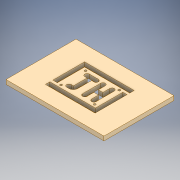
# Autodesk Inventor part: JH
Saved by Autodesk Inventor 2017 (Build 210142000, 142)
## iProperties
Created: 2016-09-28
Part Number: JH
Material: Polyethylene, High Density
Document SubType Name: Modeling
Designer: jhaun
Density: 0.952 g/cm^3
Appearance: Smooth - Off-White
Author: jhaun
Autodesk Inventor part; units mm, degrees
ref_plane "YZ Plane" through (0, 0, 0) normal (1, 0, 0) x (0, 1, 0)
ref_plane "XZ Plane" through (0, 0, 0) normal (0, 1, 0) x (-1, 0, 0)
ref_plane "XY Plane" through (0, 0, 0) normal (0, 0, 1) x (1, 0, 0)
sketch "Sketch1" plane through (0, 0, 0) normal (0, 0, 1) x (1, 0, 0)
  arc A0 (0, 6.5) -> (0, -6.5) centre (0, 0) ccw
  line L0 (0, 6.5) -> (26, 6.5)
  line L1 (0, -6.5) -> (6.5, -6.5)
  arc A1 (26, -6.5) -> (26, 6.5) centre (26, 0) ccw
  line L2 (26, -6.5) -> (19.5, -6.5)
  line L3 (6.5, -6.5) -> (6.5, -45.5)
  line L4 (19.5, -6.5) -> (19.5, -45.5)
  line L5 (6.5, -45.5) -> (0, -45.5)
  arc A2 (0, -45.5) -> (0, -58.5) centre (0, -52) ccw
  line L6 (0, -58.5) -> (6.5, -58.5)
  arc A3 (6.5, -58.5) -> (19.5, -45.5) centre (6.5, -45.5) ccw
  line L7 (39, 0) -> (39, -52)
  arc A4 (39, -52) -> (52, -52) centre (45.5, -52) ccw
  line L8 (52, -52) -> (52, -32.5)
  line L9 (52, -32.5) -> (65, -32.5)
  line L10 (65, 0) -> (65, -19.5)
  line L11 (65, -19.5) -> (52, -19.5)
  line L12 (52, -19.5) -> (52, 0)
  line L13 (78, 0) -> (78, -52)
  line L14 (65, -32.5) -> (65, -52)
  arc A5 (65, -52) -> (78, -52) centre (71.5, -52) ccw
  arc A6 (52, 0) -> (39, 0) centre (45.5, 0) ccw
  arc A7 (78, 0) -> (65, 0) centre (71.5, 0) ccw
  point P0 (0, 0)
  point P1 (0, 0)
  dimension "d0" = 26
  dimension "d1" = 6.5
  dimension "d2" = 13
  dimension "d3" = 13
  dimension "d4" = 6.5
  dimension "d5" = 13
  dimension "d6" = 39
  dimension "d7" = 39
  dimension "d8" = 6.5
  dimension "d9" = 52
  dimension "d10" = 6.5
  dimension "d11" = 13
  dimension "d12" = 19.5
  dimension "d13" = 13
  dimension "d14" = 13
  dimension "d15" = 13
  dimension "d16" = 19.5
  dimension "d17" = 13
  dimension "d19" = 52
  dimension "d20" = 13
  dimension "d22" = 6.5
  dimension "d23" = 19.5
  dimension "d24" = 6.5
  dimension "d53" = 19.5
  constraints: 30 end point, 17 point on circle, 8 centre point, 6 horizontal, 6 vertical, 1 coincident, 1 parallel
  measures "d0" distance of L0.start L0.end
  measures "d1" distance of L1.start L1.end
  measures "d2" distance between parallel lines of L1 L0
  measures "d3" distance between parallel lines of L2 L0
  measures "d4" distance of L2.start L2.end
  measures "d5" distance between parallel lines of L4 L3
  measures "d6" distance of L1.end L3.end
  measures "d7" distance of L2.end L4.end
  measures "d8" distance of L6.start A2.centre
  measures "d9" distance of L7.end L7.start
  measures "d10" distance of L7.end A4.centre
  measures "d11" distance between parallel lines of L7 L8
  measures "d12" distance of L8.start L8.end
  measures "d13" distance of L8.end L9.end
  measures "d14" distance between parallel lines of L7 L12
  measures "d15" distance between parallel lines of L11 L9
  measures "d16" distance of L11.end L12.end
  measures "d17" distance of L10.end L11.end
  measures "d19" distance of L13.start L13.end
  measures "d20" distance between parallel lines of L13 L10
  measures "d22" distance from line of point (0, 0) L0
  measures "d23" distance between parallel lines of L7 L4
  measures "d24" distance from line of point (0, 0) L3
  measures "d53" distance of L10.start L10.end
sketch "Sketch2" plane through (0, 0, 0) normal (0, 0, 1) x (1, 0, 0)
  circle A0 centre (-13.3188, 9.1594) radius 3.175
  circle A1 centre (-13.3188, -60.8406) radius 3.175
  circle A2 centre (82.6812, -60.8406) radius 3.175
  circle A3 centre (82.6812, 9.4938) radius 3.175
  line L0 (-24, 17) -> (93, 17)
  line L1 (93, 17) -> (93, -69)
  line L2 (93, -69) -> (-24, -69)
  line L3 (-24, -69) -> (-24, 17)
  line L4 (-105.5, 74) -> (174.5, 74)
  line L5 (174.5, 74) -> (174.5, -126)
  line L6 (174.5, -126) -> (-105.5, -126)
  line L7 (-105.5, -126) -> (-105.5, 74)
  line L8 (93, 9.4938) -> (105, 9.4938)
  line L9 (105, 9.4938) -> (105, -69)
  line L10 (105, -69) -> (93, -69)
  line L11 (93, -69) -> (93, 9.4938)
  line L12 (-24, -69) -> (105, -69)
  line L13 (-24, 17) -> (-24, -60.8406)
  line L14 (105, -82) -> (-37, -82)
  line L15 (-37, -82) -> (-37, -69)
  line L16 (-37, -69) -> (105, -69)
  line L17 (105, -69) -> (105, -82)
  line L18 (-24, -60.8406) -> (-37, -60.8406)
  line L19 (-37, -60.8406) -> (-37, 30)
  line L20 (-37, 30) -> (-24, 30)
  line L21 (-24, 30) -> (-24, -60.8406)
  line L22 (-24, 17) -> (105, 17)
  line L23 (105, 17) -> (105, 30)
  line L24 (105, 30) -> (-24, 30)
  line L25 (-24, 30) -> (-24, 17)
  point P0 (0, 0)
  point P1 (82.6812, 17)
  dimension "d54" = 6.35
  dimension "d55" = 6.35
  dimension "d56" = 6.35
  dimension "d57" = 6.35
  dimension "d62" = 117
  dimension "d63" = 86
  dimension "d64" = 280
  dimension "d65" = 200
  dimension "d66" = 57
  dimension "d68" = 17
  dimension "d69" = 24
  dimension "d70" = 81.5
  constraints: 52 end point, 12 parallel, 8 point on line, 7 horizontal, 6 perpendicular, 4 centre point
  measures "d54" diameter of A0
  measures "d55" diameter of A1
  measures "d56" diameter of A2
  measures "d57" diameter of A3
  measures "d62" distance of L0.end L0.start
  measures "d63" distance of L0.end L1.end
  measures "d64" distance of L4.start L4.end
  measures "d65" distance of L4.end L5.end
  measures "d66" distance between parallel lines of L4 L0
  measures "d68" distance from line of point (0, 0) L0
  measures "d69" distance from line of point (0, 0) L3
  measures "d70" distance between parallel lines of L3 L7
extrude "Extrusion6" add sketch "Sketch2" against normal blind 12 contours L0 L1 L2 L3 | L4 L5 L6 L7
extrude "Extrusion7" cut sketch "Sketch1" against normal blind 12
body "Solid4"
